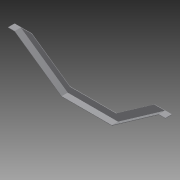
# Autodesk Inventor part: battery front L
Saved by Autodesk Inventor 2012 (Build 160160000, 160)
## iProperties
Created: 2013-10-05
Part Number: battery front L
Material: Default
Document SubType Name: Modeling
Designer: Bryce
Density: 1 g/cm^3
Author: Bryce
Autodesk Inventor part; units mm, degrees
ref_plane "YZ Plane" through (0, 0, 0) normal (1, 0, 0) x (0, 1, 0)
ref_plane "XZ Plane" through (0, 0, 0) normal (0, 1, 0) x (-1, 0, 0)
ref_plane "XY Plane" through (0, 0, 0) normal (0, 0, 1) x (1, 0, 0)
sketch "Sketch1" plane through (0, 0, 0) normal (0, 0, 1) x (1, 0, 0)
  line L0 (0, 0) -> (193.675, 0)
  line L1 (7.522, 23.8125) -> (186.153, 23.8125)
  line L2 (0, 0) -> (-180.9643, 127)
  line L3 (193.675, 0) -> (374.6393, 127)
  line L4 (-139.5115, 127) -> (7.522, 23.8125)
  line L5 (333.1865, 127) -> (186.153, 23.8125)
  line L6 (-180.9643, 127) -> (-139.5115, 127)
  line L7 (333.1865, 127) -> (374.6393, 127)
  line L8 (-181.4658, 125.4125) -> (-0.5015, -1.5875)
  line L9 (-0.5015, -1.5875) -> (194.1765, -1.5875)
  line L10 (194.1765, -1.5875) -> (375.1408, 125.4125)
  line L11 (-180.9643, 127) -> (-206.3643, 127)
  line L12 (-206.3643, 127) -> (-206.3643, 125.4125)
  line L13 (-206.3643, 125.4125) -> (-181.4658, 125.4125)
  line L14 (374.6393, 127) -> (400.0393, 127)
  line L15 (400.0393, 127) -> (400.0393, 125.4125)
  line L16 (400.0393, 125.4125) -> (375.1408, 125.4125)
  dimension "d0" = 193.675
  dimension "d1" = 23.8125
  dimension "d2" = 23.8125
  dimension "d3" = 23.8125
  dimension "d4" = 144.939
  dimension "d5" = 144.939
  dimension "d6" = 221.0816
  dimension "d7" = 221.0816
  dimension "d8" = 127
  dimension "d9" = 1.5875
  dimension "d10" = 25.4
  dimension "d11" = 1.5875
  dimension "d12" = 25.4
  dimension "d13" = 1.5875
  constraints: 34 end point, 7 parallel, 3 horizontal, 2 perpendicular, 2 other
  measures "d0" distance of L0.start L0.end
  measures "d1" distance between parallel lines of L0 L1
  measures "d2" distance between parallel lines of L2 L4
  measures "d3" distance between parallel lines of L3 L5
  measures "d4" angle of L0 L2
  measures "d5" angle of L0 L3
  measures "d6" distance of L0.start L2.end
  measures "d7" distance of L0.end L3.end
  measures "d8" vertical distance of L0.start L2.end
  measures "d9" distance between parallel lines of L9 L0
  measures "d10" distance of L2.end L11.end
  measures "d11" distance of L11.end L12.end
  measures "d12" distance of L3.end L14.end
  measures "d13" distance of L14.end L15.end
extrude "Extrusion1" add sketch "Sketch1" along normal blind 1.5875 contours L2 L6 L4 L1 L5 L7 L3 L0
extrude "Extrusion2" add sketch "Sketch1" along normal blind 25.4 contours L0 L3 L14 L15 L16 L10 L9 L8 L13 L12 L11 L2
equation "\"d2\" = d1"
equation "\"d3\" = d1"
equation "\"d4\" = d5"
equation "\"d7\" = d6"
body "Solid1"
